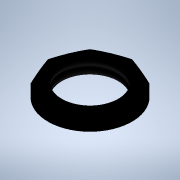
# Autodesk Inventor part: AP100_30_NUT
Saved by Autodesk Inventor 2021 (Build 250183000, 183)
## iProperties
Created: 2026-06-25
Part Number: AP100_30_NUT
Material: Generic
Catalog Web Link: www.3dfindit.com
Description: AP100 NUT-Pressure Control Valve
Vendor: SMC
Document SubType Name: Modeling
Designer: psAdmin
Manufacturer: SMC
Mass: 3.44705 g
Surface Area: 25.1261 cm^2
Volume: 3.44705 cm^3
Density: 1 g/cm^3
Appearance: PSOLRGB-0-0-0
Category: PARTsolutions
Company: SMC
Title: AP100_30_NUT
Author: Cadenas PARTsolutions
Comments: Pressure Control Valve
PSOL_IDENT_0: {$CADENAS_DATA/23d-libs/smc_jp/air_line_equipment/pressure_control_equipment/pressure_control_valve/
PSOL_IDENT_1: parts/ap100_nut.prj},167 {VTYP=3D},{NB=AP100_30_NUT},{LINA=AP100_30_NUT},{NN=AP100 NUT},{DATE=25.06.
PSOL_IDENT_2: 2026 06:59:34},{GEOMDATE=28.06.2024 09:00:00},{VERSION=},{LINEID=10},{WBVAR=},{WBNUMERIC=}  {NB=AP10
PSOL_IDENT_3: 0_30_NUT},{LINA=AP100_30_NUT},{KT=DUMMY},{RA=30}
NB: AP100_30_NUT
NN: AP100 NUT
NT: Pressure Control Valve
NBSYN: AP100_$RA._NUT
LINA: AP100_30_NUT
CATALOG: SMC (JP
RA: 30
SUPPLIER: SMC
ARTICLENO: AP100_30_NUT
BOMINFO: AP100_30_NUT
CREATOR: CADENAS GmbH
Autodesk Inventor part; units mm, degrees
sketch "Sketch_1" plane through (0, 0, 0) normal (0, 0, 1) x (1, 0, 0)
  line L0 (0, 4) -> (0, 0)
  line L1 (-23.4, 4.5573) -> (-23.4, 2)
  line L2 (-23.4, 2) -> (-19.5, 2)
  line L3 (-19.5, 2) -> (-19.5, 0)
  line L4 (-19.5, 0) -> (-13.1055, 0)
  line L5 (-13.1055, 0) -> (-13.1055, 6)
  line L6 (-13.1055, 6) -> (-18.0157, 6)
  line L7 (-18.0157, 6) -> (-23.4, 4.5573)
  constraints: 16 end point
revolve "Revolution1" add sketch "Sketch_1" angle 360 about axis through (0, 4, 0) along (0, 1, 0)
thread "Thread1" size "M30x3.5" class "6H" standard "ISO Metric profile" full length
sketch "Sketch_4" plane through (0, 2, 0) normal (0, 1, 0) x (1, 0, 0)
  circle A0 centre (0, 0) radius 50
  line L0 (-19.5, 0) -> (-13.7886, -13.7886)
  line L1 (-13.7886, -13.7886) -> (0, -19.5)
  line L2 (0, -19.5) -> (13.7886, -13.7886)
  line L3 (13.7886, -13.7886) -> (19.5, 0)
  line L4 (19.5, 0) -> (13.7886, 13.7886)
  line L5 (13.7886, 13.7886) -> (0, 19.5)
  line L6 (0, 19.5) -> (-13.7886, 13.7886)
  line L7 (-13.7886, 13.7886) -> (-19.5, 0)
  constraints: 16 end point, 1 centre point
extrude "Extrusion1" cut sketch "Sketch_4" along normal blind 4
ref_plane "nut_body_XY" through (0, 0, 0) normal (0, -1, 0) x (1, 0, 0)
ref_plane "nut_body_YZ" through (0, 0, 0) normal (1, 0, 0) x (0, 0, 1)
ref_plane "nut_body_ZX" through (0, 0, 0) normal (0, 0, 1) x (0, -1, 0)
body "Solid1"
